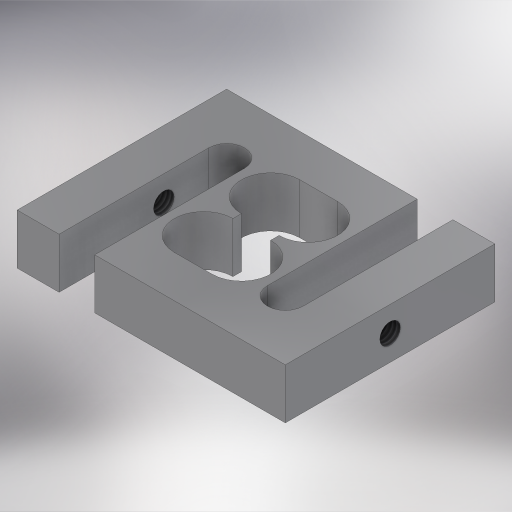
# Autodesk Inventor part: Célula de carga
Saved by Autodesk Inventor 2023 (Build 270158000, 158)
## iProperties
Created: 2023-03-17
Part Number: Célula de carga
Material: Alumínio 6061
Document SubType Name: Sheet Metal
Designer: Mateus
Density: 2.7 g/cm^3
Sheet Metal Rule: Padrão_mm
Appearance: Alumínio - Polido
Mass: 62.4013 g
Surface Area: 100.363 cm^2
Volume: 23.1116 cm^3
Author: Mateus
Autodesk Inventor part; units mm, degrees
ref_plane "YZ Plane" through (0, 0, 0) normal (1, 0, 0) x (0, 1, 0)
ref_plane "XZ Plane" through (0, 0, 0) normal (0, 1, 0) x (-1, 0, 0)
ref_plane "XY Plane" through (0, 0, 0) normal (0, 0, 1) x (1, 0, 0)
sketch "Esboço1" plane through (0, 0, 0) normal (0, 1, 0) x (-1, 0, 0)
  line L0 (0, 0) -> (45.5, 0)
  line L1 (45.5, 0) -> (45.5, -35.75)
  line L2 (49.75, -40) -> (49.75, -40)
  line L3 (54, -35.75) -> (54, 0)
  line L4 (54, 0) -> (64, 0)
  line L5 (64, 0) -> (64, -50)
  line L6 (64, -50) -> (18.5, -50)
  line L7 (18.5, -50) -> (18.5, -14.25)
  line L8 (14.25, -10) -> (14.25, -10)
  line L9 (10, -14.25) -> (10, -50)
  line L10 (10, -50) -> (0, -50)
  line L11 (0, -50) -> (0, 0)
  arc A0 (18.5, -14.25) -> (14.25, -10) centre (14.25, -14.25) ccw
  arc A1 (14.25, -10) -> (10, -14.25) centre (14.25, -14.25) ccw
  arc A2 (45.5, -35.75) -> (49.75, -40) centre (49.75, -35.75) ccw
  arc A3 (49.75, -40) -> (54, -35.75) centre (49.75, -35.75) ccw
  point P0 (45.5, -40)
  point P1 (54, -40)
  point P2 (10, -10)
  dimension "d0" = 64
  dimension "d1" = 10
  dimension "d2" = 40
  dimension "d3" = 50
  dimension "d4" = 8.5
  dimension "d5" = 4.25
  constraints: 24 end point, 10 point on line, 9 perpendicular, 8 point on circle, 8 tangent, 4 centre point, 3 equal radius, 3 parallel, 1 horizontal
  measures "d0" distance of L0.start L4.end
  measures "d1" distance of L9.end L10.end
  measures "d2" distance of point (10, -10) L9.end
  measures "d3" distance of L10.end L0.start
  measures "d4" distance of point (45.5, -40) point (54, -40)
  measures "d5" radius of A0
extrude "Extrusão1" add sketch "Esboço1" along normal blind 12
sketch "Esboço2" plane through (0, 0, 0) normal (1, 0, 0) x (0, 0, -1)
  line L0 (0, 12) -> (50, 12) projected
  line L1 (50, 0) -> (50, 12) projected
  point P0 (0, 0)
  point P1 (25, 6)
  dimension "d8" = 50
  dimension "d9" = 12
  dimension "d10" = 6
  dimension "d11" = 25
  measures "d8" distance of L0.start L0.end
  measures "d9" distance of L1.start L0.end
  measures "d10" distance from line of L0 point (25, 6)
  measures "d11" distance from line of L1 point (25, 6)
hole "Furo1" at (0, 6, -25) direction (-1, 0, 0) diameter 4.917 depth 10 thread size "M6x1" class "6H" standard "ISO Metric profile"
sketch "Esboço3" plane through (-64, 0, -50) normal (-1, 0, 0) x (0, 0, 1)
  line L0 (0, 0) -> (50, 0) projected
  line L1 (0, 0) -> (0, 12) projected
  circle A0 centre (25, 6) radius 2.4585 projected
  dimension "d19" = 50
  dimension "d20" = 12
  constraints: 1 coincident
  measures "d19" distance of L0.start L0.end
  measures "d20" distance of L0.start L1.end
hole "Furo2" at (-64, 6, -25) direction (1, 0, 0) diameter 4.917 depth 10 thread size "M6x1" class "6H" standard "ISO Metric profile"
sketch "Sketch4" plane through (0, 12, 0) normal (0, 1, 0) x (1, 0, 0)
  line L0 (-36.5, 10) -> (-27.4995, 10)
  arc A0 (-27.4995, 10) -> (-27.4995, 24) centre (-27.4995, 17) ccw
  arc A1 (-36.5002, 24) -> (-36.5, 10) centre (-36.5, 17) ccw
  line L1 (-36.5, 24) -> (-27.4995, 24)
  line L2 (-13.5, 10) -> (-19.5, 10) projected
  line L3 (-36.5002, 26.001) -> (-27.4998, 26.001)
  arc A2 (-27.4998, 26.001) -> (-27.6165, 40) centre (-27.4998, 33.001) ccw
  arc A3 (-36.6169, 40) -> (-36.5002, 26.001) centre (-36.5002, 33.001) ccw
  line L4 (-36.6169, 40) -> (-27.6165, 40)
  line L5 (-45.5, 35.75) -> (-45.5, 0) projected
  line L6 (-50.5, 40) -> (-44.5, 40) projected
  line L7 (-18.5, 14.25) -> (-18.5, 50) projected
  line L8 (-36.5002, 26.001) -> (-27.4995, 26.001)
  line L9 (-27.4995, 26.001) -> (-27.4995, 24)
  line L10 (-27.4995, 24) -> (-36.5002, 24)
  line L11 (-36.5002, 24) -> (-36.5002, 26.001)
  point P0 (0, 0)
  point P1 (-31.9998, 10)
  point P2 (-20.5, 33.0593)
  point P3 (-43.5, 32.9426)
  point P4 (-32, 26.001)
  point P5 (-43.5, 16.9999)
  dimension "d28" = 0
  dimension "d29" = 0
  dimension "d30" = 23
  dimension "d31" = 13.5
  dimension "d32" = 27
  dimension "d33" = 0
  dimension "d34" = 7
  dimension "d35" = 0
  constraints: 16 end point, 11 point on circle, 5 parallel, 5 tangent, 4 centre point, 4 horizontal, 2 equal radius, 2 midpoint, 2 perpendicular
  measures "d28" distance from line of L2 point (-32, 10)
  measures "d29" distance between parallel lines of L6 L4
  measures "d30" horizontal distance of point (-20.5, 33.059) point (-43.5, 32.943)
  measures "d31" distance from line of L7 point (-32, 26.001)
  measures "d32" distance between parallel lines of L7 L5
  measures "d33" horizontal distance of A1.start L3.start
  measures "d34" radius of A2
  measures "d35" horizontal distance of point (-43.5, 17) point (-43.5, 32.943)
extrude "Extrusion2" cut sketch "Sketch4" against normal through all
equation "\"d10\" = 0.5 * d9"
equation "\"d11\" = 0.5 * d8"
equation "\"d17\" = Espessura"
equation "\"d31\" = 0.5 * d32"
equation "\"Raio_vergadura\" = Espessura"
equation "\"Largura_alívio_de_vergadura\" = Espessura"
equation "\"Profundidade_alívio_de_vergadura\" = 0.5 * Espessura"
equation "\"Tamanho_alívio_de_dobra\" = 4 * Espessura"
equation "\"Remanescente_mínimo\" = 2 * Espessura"
equation "\"Raiodetransição\" = Raio_vergadura"
equation "\"Tamanho_de_raio_de_Jacobi\" = Raio_vergadura"
equation "\"TamanhoFolga\" = Espessura"
equation "\"Espessura\" = 0.5"
